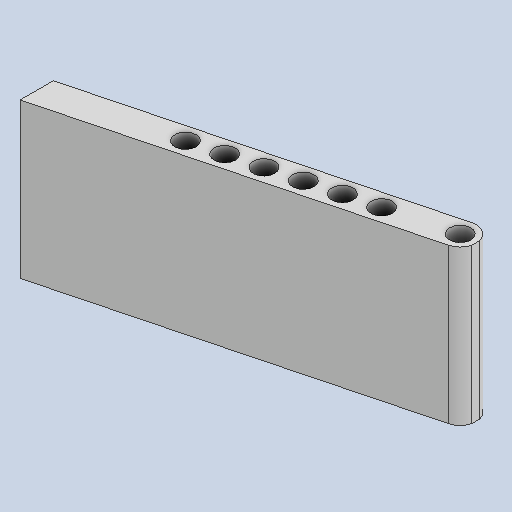
# Autodesk Inventor part: only_top_gate
Saved by Autodesk Inventor 2025.2 (Build 292293000, 293)
## iProperties
Created: 2025-01-19
Part Number: only_top_gate
Material: Типовые
Document SubType Name: Modeling
Designer: Admin
Density: 1 g/cm^3
Appearance: По умолчанию
Author: Admin
Autodesk Inventor part; units mm, degrees
ref_plane "YZ Plane" through (0, 0, 0) normal (1, 0, 0) x (0, 1, 0)
ref_plane "XZ Plane" through (0, 0, 0) normal (0, 1, 0) x (-1, 0, 0)
ref_plane "XY Plane" through (0, 0, 0) normal (0, 0, 1) x (1, 0, 0)
sketch "Эскиз1" plane through (0, 0, 0) normal (0, 1, 0) x (-1, 0, 0)
  line L0 (-53.5804, -13.9309) -> (-0.75, -0.195)
  line L1 (-52.3223, -18.77) -> (-0.75, -5.3612)
  line L2 (-55.3709, -15.7214) -> (-55.3709, -16.9796)
  circle A0 centre (-52.9514, -16.3505) radius 1.65
  line L3 (-0.75, -5.3612) -> (-0.75, -0.195)
  arc A1 (-55.3709, -16.9796) -> (-52.3223, -18.77) centre (-52.9514, -16.3505) ccw
  arc A2 (-53.5804, -13.9309) -> (-55.3709, -15.7214) centre (-52.9514, -16.3505) ccw
  point P0 (0, 0)
  constraints: 8 end point, 4 point on circle, 3 centre point, 1 coincident
extrude "Выдавливание1" add sketch "Эскиз1" along normal blind 24
sketch "Эскиз24" plane through (0, 24, 0) normal (0, 1, 0) x (1, 0, 0)
  circle A0 centre (52.9514, 16.3505) radius 1.65 projected
  line L0 (52.9514, 16.3505) -> (43.2731, 13.8341)
  circle A1 centre (43.2731, 13.8341) radius 1.65
  circle A2 centre (38.434, 12.576) radius 1.65
  line L1 (48.1122, 15.0923) -> (38.434, 12.576)
  circle A3 centre (33.5949, 11.3178) radius 1.65
  line L2 (43.2731, 13.8341) -> (33.5949, 11.3178)
  circle A4 centre (28.7558, 10.0596) radius 1.65
  line L3 (38.434, 12.576) -> (28.7558, 10.0596)
  circle A5 centre (23.9167, 8.8015) radius 1.65
  line L4 (33.5949, 11.3178) -> (23.9167, 8.8015)
  circle A6 centre (19.0776, 7.5433) radius 1.65
  line L5 (28.7558, 10.0596) -> (19.0776, 7.5433)
  point P0 (0, 0)
  dimension "d126" = 3.3
  dimension "d129" = 5
  constraints: 12 end point, 6 centre point, 6 coincident, 1 collinear, 25 other
  measures "d126" diameter of A1
  measures "d129" distance of A1.centre A2.centre
extrude "Выдавливание24" cut sketch "Эскиз24" against normal blind 3 contours A6 | A5 L5 L4 | L4 L5 A5 | A4 L4 L3 | L3 L4 A4 | A3 L3 L2 | L2 L3 A3 | A2 L2 L1 | L1 L2 A2 | A1 L1 L0 | L0 L1 A1
sketch "Эскиз25" plane through (19.0776, 21, -7.5433) normal (0, 1, 0) x (1, 0, 0)
  circle A0 centre (0, 0) radius 1.65 projected
  circle A1 centre (0, 0) radius 1.15
  circle A2 centre (4.8391, 1.2582) radius 1.65 projected
  circle A3 centre (4.8391, 1.2582) radius 1.15
  circle A4 centre (9.6782, 2.5163) radius 1.65 projected
  circle A5 centre (9.6782, 2.5163) radius 1.15
  circle A6 centre (14.5173, 3.7745) radius 1.65 projected
  circle A7 centre (14.5173, 3.7745) radius 1.15
  circle A8 centre (19.3565, 5.0327) radius 1.65 projected
  circle A9 centre (19.3565, 5.0327) radius 1.15
  circle A10 centre (24.1956, 6.2908) radius 1.65 projected
  circle A11 centre (24.1956, 6.2908) radius 1.15
  point P0 (-19.0776, -7.5433)
  dimension "d136" = 2.3
  dimension "d137" = 2.3
  dimension "d138" = 2.3
  dimension "d139" = 2.3
  dimension "d140" = 2.3
  dimension "d141" = 2.3
  constraints: 6 centre point, 6 coincident
  measures "d136" diameter of A1
  measures "d137" diameter of A3
  measures "d138" diameter of A5
  measures "d139" diameter of A7
  measures "d140" diameter of A9
  measures "d141" diameter of A11
extrude "Выдавливание25" cut sketch "Эскиз25" against normal blind 5 contours A1 | A3 | A5 | A7 | A9 | A11
